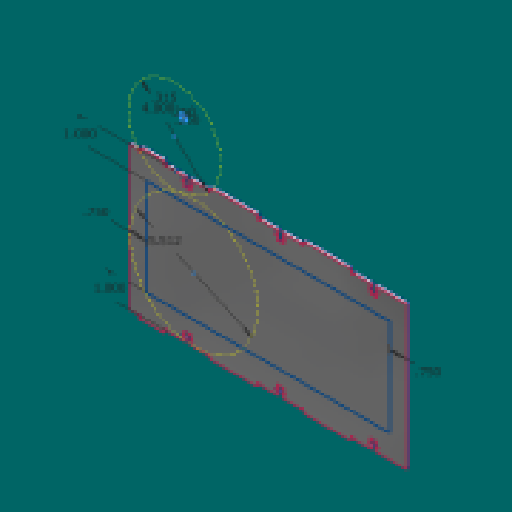
# Autodesk Inventor part: ConveyorSlide
Saved by Autodesk Inventor 2023.1 (Build 271208000, 208)
## iProperties
Created: 2022-11-11
Part Number: ConveyorSlide
Material: Aluminum 6061
Document SubType Name: Modeling
Designer: zac-h
Density: 2.7 g/cm^3
Appearance: Aluminum - Flat
Author: zac-h
Autodesk Inventor part; units mm, degrees
ref_plane "YZ Plane" through (0, 0, 0) normal (1, 0, 0) x (0, 1, 0)
ref_plane "XZ Plane" through (0, 0, 0) normal (0, 1, 0) x (-1, 0, 0)
ref_plane "XY Plane" through (0, 0, 0) normal (0, 0, 1) x (1, 0, 0)
ref_plane "Work Plane1" through (0, 0, 0) normal (0, 0, 1) x (1, 0, 0)
sketch "Sketch1" plane through (0, 0, 0) normal (0, 0, 1) x (1, 0, 0)
  line L0 (0, 0) -> (25.4, 0) projected
  line L1 (25.4, 0) -> (25.4, 3) projected
  line L2 (0, 3) -> (25.4, 3) construction
  line L3 (0, 0) -> (0, 3) projected
  line L4 (48.641, 3) -> (52.959, 3) construction
  line L5 (76.2, 0) -> (127, 0) projected
  line L6 (127, 0) -> (127, 3) projected
  line L7 (76.2, 3) -> (127, 3) construction
  line L8 (76.2, 0) -> (76.2, 3) projected
  line L9 (150.241, 3) -> (154.559, 3) construction
  line L10 (177.8, 0) -> (228.6, 0) projected
  line L11 (228.6, 0) -> (228.6, 3) projected
  line L12 (177.8, 3) -> (228.6, 3) construction
  line L13 (177.8, 0) -> (177.8, 3) projected
  line L14 (251.841, 3) -> (256.159, 3) construction
  line L15 (256.159, 3) -> (256.159, 6)
  line L16 (256.159, 6) -> (258.064, 6)
  line L17 (258.064, 6) -> (258.064, 12.858)
  line L18 (258.064, 12.858) -> (249.936, 12.858)
  line L19 (249.936, 12.858) -> (249.936, 6)
  line L20 (249.936, 6) -> (251.841, 6)
  line L21 (251.841, 6) -> (251.841, 3)
  line L22 (256.159, 3) -> (290.449, 3)
  line L23 (290.449, 3) -> (290.449, 81.28)
  line L24 (-255.6541, 81.28) -> (660.8228, 81.28)
  line L25 (251.841, 3) -> (228.6, 3)
  line L26 (177.8, 3) -> (154.559, 3)
  line L27 (154.559, 3) -> (154.559, 6)
  line L28 (154.559, 6) -> (156.464, 6)
  line L29 (156.464, 6) -> (156.464, 12.858)
  line L30 (156.464, 12.858) -> (148.336, 12.858)
  line L31 (148.336, 12.858) -> (148.336, 6)
  line L32 (148.336, 6) -> (150.241, 6)
  line L33 (150.241, 6) -> (150.241, 3)
  line L34 (150.241, 3) -> (127, 3)
  line L35 (76.2, 3) -> (52.959, 3)
  line L36 (52.959, 3) -> (52.959, 6)
  line L37 (52.959, 6) -> (54.864, 6)
  line L38 (54.864, 6) -> (54.864, 12.858)
  line L39 (54.864, 12.858) -> (46.736, 12.858)
  line L40 (46.736, 12.858) -> (46.736, 6)
  line L41 (46.736, 6) -> (48.641, 6)
  line L42 (48.641, 6) -> (48.641, 3)
  line L43 (48.641, 3) -> (25.4, 3)
  line L44 (0, 3) -> (-12.7, 3)
  line L45 (-12.7, 3) -> (-12.7, 81.28)
  circle A0 centre (258.064, 7.75) radius 1.75
  circle A1 centre (256.8266, 11.6206) radius 1.75
  line L46 (256.8266, 11.6206) -> (258.064, 12.858) construction
  line L47 (254, 3) -> (254, 12.858) construction
  circle A2 centre (249.936, 7.75) radius 1.75
  circle A3 centre (251.1734, 11.6206) radius 1.75
  line L48 (156.464, 12.858) -> (155.2266, 11.6206) construction
  circle A4 centre (155.2266, 11.6206) radius 1.75
  circle A5 centre (156.464, 7.75) radius 1.75
  line L49 (152.4, 3) -> (152.4, 12.858) construction
  circle A6 centre (149.5734, 11.6206) radius 1.75
  circle A7 centre (148.336, 7.75) radius 1.75
  line L50 (54.864, 12.858) -> (53.6266, 11.6206) construction
  circle A8 centre (53.6266, 11.6206) radius 1.75
  circle A9 centre (54.864, 7.75) radius 1.75
  line L51 (50.8, 3) -> (50.8, 12.858) construction
  circle A10 centre (47.9734, 11.6206) radius 1.75
  circle A11 centre (46.736, 7.75) radius 1.75
  circle A12 centre (128.75, 3) radius 1.75
  circle A13 centre (74.45, 3) radius 1.75
  circle A14 centre (27.15, 3) radius 1.75
  circle A15 centre (-1.75, 3) radius 1.75
  circle A16 centre (176.05, 3) radius 1.75
  circle A17 centre (230.35, 3) radius 1.75
  point P0 (46.736, 9.5)
  point P1 (46.736, 10.3831)
  point P2 (49.2109, 12.858)
  point P3 (52.3891, 12.858)
  point P4 (54.864, 10.3831)
  point P5 (54.864, 9.5)
  point P6 (148.336, 9.5)
  point P7 (148.336, 10.3831)
  point P8 (150.8109, 12.858)
  point P9 (153.9891, 12.858)
  point P10 (156.464, 10.3831)
  point P11 (156.464, 9.5)
  point P12 (249.936, 6)
  point P13 (249.936, 9.5)
  point P14 (249.936, 10.3831)
  point P15 (252.4109, 12.858)
  point P16 (255.5891, 12.858)
  point P17 (258.064, 10.3831)
  point P18 (258.064, 9.5)
  point P19 (28.9, 3)
  point P20 (72.7, 3)
  point P21 (130.5, 3)
  point P22 (174.3, 3)
  point P23 (232.1, 3)
  point P24 (-3.5, 3)
  dimension "d11" = 3.5
  dimension "d14" = 3.5
  dimension "d16" = 3.5
  dimension "d17" = 3.5
  dimension "d0" = 3
  dimension "d1" = 8.128
  dimension "d2" = 6.858
  dimension "d3" = 34.29
  dimension "d6" = 3
  dimension "d7" = 3
  dimension "d8" = 12.7
  dimension "d12" = 45
  dimension "d13" = 45
  dimension "d15" = 45
  constraints: 74 end point, 16 perpendicular, 15 point on line, 7 equal length, 7 horizontal, 6 centre point, 6 midpoint, 6 symmetric about line, 5 vertical, 2 coincident, 2 collinear, 44 other
  measures "d0" distance of L14.end L15.end
  measures "d1" distance between parallel lines of L17 L19
  measures "d2" distance of L16.end L17.end
  measures "d3" distance of L14.end L22.end
  measures "d6" distance of L32.end L9.start
  measures "d7" distance of L4.end L36.end
  measures "d8" distance of L2.start L44.end
  measures "d12" angle of L18 L46
  measures "d13" angle of L30 L48
  measures "d15" angle of L39 L50
extrude "Extrusion1" add sketch "Sketch1" along normal blind 3 contours L3 A15 L44 L45 L24 L23 L22 L15 L16 A0 L17 A1 L18 A3 L19 A2 L20 L21 L25 A17 L11 L10 L13 A16 L26 L27 L28 A5 L29 A4 L30 A6 L31 A7 L32 L33 L34 A12 L6 L5 L8 A13 L35 L36 L37 A9 L38 A8 L39 A10 L40 A11 L41 L42 L43 A14 L1 L0
mirror "Mirror1" about plane through (290.449, 81.28, 0) normal (0, 1, 0) of "Extrusion1"
sketch "Sketch2" plane through (0, 0, 3) normal (0, 0, 1) x (1, 0, 0)
  line L0 (0, 0) -> (25.4, 0) projected
  line L1 (25.4, 0) -> (25.4, 3) projected
  arc A0 (28.9, 3) -> (25.4, 3) centre (27.15, 3) ccw projected
  line L2 (28.9, 3) -> (48.641, 3) projected
  line L3 (48.641, 3) -> (48.641, 6) projected
  line L4 (48.641, 6) -> (46.736, 6) projected
  arc A1 (46.736, 9.5) -> (46.736, 6) centre (46.736, 7.75) ccw projected
  line L5 (46.736, 9.5) -> (46.736, 10.3831) projected
  arc A2 (49.2109, 12.858) -> (46.736, 10.3831) centre (47.9734, 11.6206) ccw projected
  line L6 (49.2109, 12.858) -> (52.3891, 12.858) projected
  arc A3 (54.864, 10.3831) -> (52.3891, 12.858) centre (53.6266, 11.6206) ccw projected
  line L7 (54.864, 10.3831) -> (54.864, 9.5) projected
  arc A4 (54.864, 6) -> (54.864, 9.5) centre (54.864, 7.75) ccw projected
  line L8 (54.864, 6) -> (52.959, 6) projected
  line L9 (52.959, 6) -> (52.959, 3) projected
  line L10 (52.959, 3) -> (72.7, 3) projected
  arc A5 (76.2, 3) -> (72.7, 3) centre (74.45, 3) ccw projected
  line L11 (76.2, 3) -> (76.2, 0) projected
  line L12 (76.2, 0) -> (127, 0) projected
  line L13 (127, 0) -> (127, 3) projected
  arc A6 (130.5, 3) -> (127, 3) centre (128.75, 3) ccw projected
  line L14 (130.5, 3) -> (150.241, 3) projected
  line L15 (150.241, 3) -> (150.241, 6) projected
  line L16 (150.241, 6) -> (148.336, 6) projected
  arc A7 (148.336, 9.5) -> (148.336, 6) centre (148.336, 7.75) ccw projected
  line L17 (148.336, 9.5) -> (148.336, 10.3831) projected
  arc A8 (150.8109, 12.858) -> (148.336, 10.3831) centre (149.5734, 11.6206) ccw projected
  line L18 (150.8109, 12.858) -> (153.9891, 12.858) projected
  arc A9 (156.464, 10.3831) -> (153.9891, 12.858) centre (155.2266, 11.6206) ccw projected
  line L19 (156.464, 10.3831) -> (156.464, 9.5) projected
  arc A10 (156.464, 6) -> (156.464, 9.5) centre (156.464, 7.75) ccw projected
  line L20 (156.464, 6) -> (154.559, 6) projected
  line L21 (154.559, 6) -> (154.559, 3) projected
  line L22 (154.559, 3) -> (174.3, 3) projected
  arc A11 (177.8, 3) -> (174.3, 3) centre (176.05, 3) ccw projected
  line L23 (177.8, 3) -> (177.8, 0) projected
  line L24 (177.8, 0) -> (228.6, 0) projected
  line L25 (228.6, 0) -> (228.6, 3) projected
  arc A12 (232.1, 3) -> (228.6, 3) centre (230.35, 3) ccw projected
  line L26 (232.1, 3) -> (251.841, 3) projected
  line L27 (251.841, 3) -> (251.841, 6) projected
  line L28 (251.841, 6) -> (249.936, 6) projected
  arc A13 (249.936, 9.5) -> (249.936, 6) centre (249.936, 7.75) ccw projected
  line L29 (249.936, 9.5) -> (249.936, 10.3831) projected
  arc A14 (252.4109, 12.858) -> (249.936, 10.3831) centre (251.1734, 11.6206) ccw projected
  line L30 (252.4109, 12.858) -> (255.5891, 12.858) projected
  arc A15 (258.064, 10.3831) -> (255.5891, 12.858) centre (256.8266, 11.6206) ccw projected
  line L31 (258.064, 10.3831) -> (258.064, 9.5) projected
  arc A16 (258.064, 6) -> (258.064, 9.5) centre (258.064, 7.75) ccw projected
  line L32 (258.064, 6) -> (256.159, 6) projected
  line L33 (256.159, 6) -> (256.159, 3) projected
  line L34 (256.159, 3) -> (290.449, 3) projected
  line L35 (290.449, 3) -> (290.449, 159.56) projected
  line L36 (256.159, 159.56) -> (290.449, 159.56) projected
  line L37 (256.159, 156.56) -> (256.159, 159.56) projected
  line L38 (258.064, 156.56) -> (256.159, 156.56) projected
  arc A17 (258.064, 153.06) -> (258.064, 156.56) centre (258.064, 154.81) ccw projected
  line L39 (258.064, 152.1769) -> (258.064, 153.06) projected
  arc A18 (255.5891, 149.702) -> (258.064, 152.1769) centre (256.8266, 150.9394) ccw projected
  line L40 (252.4109, 149.702) -> (255.5891, 149.702) projected
  arc A19 (249.936, 152.1769) -> (252.4109, 149.702) centre (251.1734, 150.9394) ccw projected
  line L41 (249.936, 153.06) -> (249.936, 152.1769) projected
  arc A20 (249.936, 156.56) -> (249.936, 153.06) centre (249.936, 154.81) ccw projected
  line L42 (251.841, 156.56) -> (249.936, 156.56) projected
  line L43 (251.841, 159.56) -> (251.841, 156.56) projected
  line L44 (232.1, 159.56) -> (251.841, 159.56) projected
  arc A21 (228.6, 159.56) -> (232.1, 159.56) centre (230.35, 159.56) ccw projected
  line L45 (228.6, 162.56) -> (228.6, 159.56) projected
  line L46 (177.8, 162.56) -> (228.6, 162.56) projected
  line L47 (177.8, 159.56) -> (177.8, 162.56) projected
  arc A22 (174.3, 159.56) -> (177.8, 159.56) centre (176.05, 159.56) ccw projected
  line L48 (154.559, 159.56) -> (174.3, 159.56) projected
  line L49 (154.559, 156.56) -> (154.559, 159.56) projected
  line L50 (156.464, 156.56) -> (154.559, 156.56) projected
  arc A23 (156.464, 153.06) -> (156.464, 156.56) centre (156.464, 154.81) ccw projected
  line L51 (156.464, 152.1769) -> (156.464, 153.06) projected
  arc A24 (153.9891, 149.702) -> (156.464, 152.1769) centre (155.2266, 150.9394) ccw projected
  line L52 (150.8109, 149.702) -> (153.9891, 149.702) projected
  arc A25 (148.336, 152.1769) -> (150.8109, 149.702) centre (149.5734, 150.9394) ccw projected
  line L53 (148.336, 153.06) -> (148.336, 152.1769) projected
  arc A26 (148.336, 156.56) -> (148.336, 153.06) centre (148.336, 154.81) ccw projected
  line L54 (150.241, 156.56) -> (148.336, 156.56) projected
  line L55 (150.241, 159.56) -> (150.241, 156.56) projected
  line L56 (130.5, 159.56) -> (150.241, 159.56) projected
  arc A27 (127, 159.56) -> (130.5, 159.56) centre (128.75, 159.56) ccw projected
  line L57 (127, 162.56) -> (127, 159.56) projected
  line L58 (76.2, 162.56) -> (127, 162.56) projected
  line L59 (76.2, 159.56) -> (76.2, 162.56) projected
  arc A28 (72.7, 159.56) -> (76.2, 159.56) centre (74.45, 159.56) ccw projected
  line L60 (52.959, 159.56) -> (72.7, 159.56) projected
  line L61 (52.959, 156.56) -> (52.959, 159.56) projected
  line L62 (54.864, 156.56) -> (52.959, 156.56) projected
  arc A29 (54.864, 153.06) -> (54.864, 156.56) centre (54.864, 154.81) ccw projected
  line L63 (54.864, 152.1769) -> (54.864, 153.06) projected
  arc A30 (52.3891, 149.702) -> (54.864, 152.1769) centre (53.6266, 150.9394) ccw projected
  line L64 (49.2109, 149.702) -> (52.3891, 149.702) projected
  arc A31 (46.736, 152.1769) -> (49.2109, 149.702) centre (47.9734, 150.9394) ccw projected
  line L65 (46.736, 153.06) -> (46.736, 152.1769) projected
  arc A32 (46.736, 156.56) -> (46.736, 153.06) centre (46.736, 154.81) ccw projected
  line L66 (48.641, 156.56) -> (46.736, 156.56) projected
  line L67 (48.641, 159.56) -> (48.641, 156.56) projected
  line L68 (28.9, 159.56) -> (48.641, 159.56) projected
  arc A33 (25.4, 159.56) -> (28.9, 159.56) centre (27.15, 159.56) ccw projected
  line L69 (25.4, 162.56) -> (25.4, 159.56) projected
  line L70 (0, 162.56) -> (25.4, 162.56) projected
  line L71 (0, 159.56) -> (0, 162.56) projected
  arc A34 (-3.5, 159.56) -> (0, 159.56) centre (-1.75, 159.56) ccw projected
  line L72 (-12.7, 159.56) -> (-3.5, 159.56) projected
  line L73 (-12.7, 3) -> (-12.7, 159.56) projected
  line L74 (-12.7, 3) -> (-3.5, 3) projected
  arc A35 (0, 3) -> (-3.5, 3) centre (-1.75, 3) ccw projected
  line L75 (0, 3) -> (0, 0) projected
  line L76 (6.35, 28.4) -> (271.399, 28.4)
  line L77 (271.399, 28.4) -> (271.399, 134.16)
  line L78 (271.399, 134.16) -> (6.35, 134.16)
  line L79 (6.35, 134.16) -> (6.35, 28.4)
  circle A36 centre (58.2545, 73) radius 70 construction
  line L80 (28.9, 3) -> (48.641, 3) projected
  circle A37 centre (37.2332, 191.5885) radius 50.8 construction
  circle A38 centre (45.9692, 213.8681) radius 4
  line L81 (42.7942, 210.6931) -> (49.1442, 210.6931)
  line L82 (49.1442, 210.6931) -> (49.1442, 217.0431)
  line L83 (49.1442, 217.0431) -> (42.7942, 217.0431)
  line L84 (42.7942, 217.0431) -> (42.7942, 210.6931)
  line L85 (42.7942, 210.6931) -> (49.1442, 217.0431) construction
  line L86 (49.1442, 210.6931) -> (42.7942, 217.0431) construction
  point P0 (38.7705, 159.56)
  dimension "d18" = 19.05
  dimension "d19" = 25.4
  dimension "d20" = 25.4
  dimension "d21" = 19.05
  dimension "d22" = 140
  dimension "d23" = 101.6
  dimension "d24" = 8
  dimension "d25" = 6.35
  dimension "d26" = 6.35
  constraints: 20 end point, 4 parallel, 3 centre point, 3 midpoint, 2 horizontal, 2 perpendicular, 1 tangent
  measures "d18" distance between parallel lines of L73 L79
  measures "d19" distance between parallel lines of L2 L76
  measures "d20" distance from line of point (38.771, 159.56) L78
  measures "d21" distance between parallel lines of L35 L77
  measures "d22" diameter of A36
  measures "d23" diameter of A37
  measures "d24" diameter of A38
  measures "d25" distance of L83.end L82.end
  measures "d26" distance of L82.end L81.end
body "Solid1"
